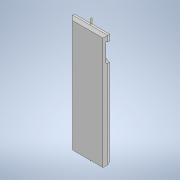
# Autodesk Inventor part: Part3
Saved by Autodesk Inventor 2022 (Build 260153000, 153)
## iProperties
Created: 2020-04-25
Part Number: Part3
Material: Generic
Document SubType Name: Modeling
Designer: Martijn
Density: 1 g/cm^3
Appearance: Default
Author: Martijn
Autodesk Inventor part; units mm, degrees
ref_plane "YZ Plane" through (0, 0, 0) normal (1, 0, 0) x (0, 1, 0)
ref_plane "XZ Plane" through (0, 0, 0) normal (0, 1, 0) x (-1, 0, 0)
ref_plane "XY Plane" through (0, 0, 0) normal (0, 0, 1) x (1, 0, 0)
sketch "Sketch1" plane through (0, 0, 0) normal (0, 0, 1) x (1, 0, 0)
  line L0 (0, 0) -> (24.6, 0)
  line L1 (24.6, 0) -> (24.6, 80.1)
  line L2 (24.6, 80.1) -> (0, 80.1)
  line L3 (0, 80.1) -> (0, 0)
  dimension "d0" = 24.6
  dimension "d18" = 80.1
  constraints: 8 end point, 2 perpendicular, 1 horizontal
  measures "d0" distance between parallel lines of L3 L1
  measures "d18" distance between parallel lines of L2 L0
extrude "Extrusion1" add sketch "Sketch1" along normal blind 3
chamfer "Chamfer1" distance 1.7 angle 45 3 edges at (0, 40.05, 3) (24.6, 40.05, 3) (12.3, 80.1, 3)
chamfer "Chamfer2" distance 3 angle 45 1 edges at (12.3, 0, 0)
sketch "Sketch3" plane through (0, 0, 0) normal (0, 0, -1) x (-1, 0, 0)
  arc A0 (-30.6, 63.1) -> (-17.6, 76.1) centre (-27.6, 73.1) ccw
  line L0 (-24.6, 80.1) -> (0, 80.1) projected
  line L1 (-24.6, 3) -> (-24.6, 80.1) projected
  line L2 (-17.6, 76.1) -> (-30.6, 76.1)
  line L3 (-30.6, 76.1) -> (-30.6, 63.1)
  point P0 (0, 0)
  dimension "d19" = 7
  dimension "d20" = 3
  dimension "d21" = 3
  dimension "d22" = 3
  dimension "d23" = 13
  constraints: 4 end point, 2 point on circle, 1 centre point, 1 horizontal, 1 perpendicular
  measures "d19" distance from line of L0 A0.centre
  measures "d20" distance from line of L1 A0.centre
  measures "d21" horizontal distance of L3.end A0.centre
  measures "d22" vertical distance of A0.centre L2.start
  measures "d23" distance of L2.end L3.end
extrude "Extrusion3" cut sketch "Sketch3" against normal blind 2
ref_plane "Work Plane1" through (12.3, 3, 0) normal (-1, 0, 0) x (0, 0, 1)
mirror "Mirror1" about plane through (12.3, 3, 0) normal (-1, 0, 0) of "Extrusion3"
ref_plane "Work Plane2" through (12.3, 3, 0) normal (-1, 0, 0) x (0, 0, 1)
body "Solid1"
